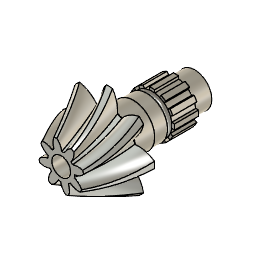
SanmitraGoswami helical bevel gear (Autodesk Fusion 360 design; units mm, degrees)
part number: 2025-10-19-15-40-55-736
Autodesk Fusion 360 part; units mm, degrees
sketch "Sketch2" plane through (0, 0, 0) normal (1, 0, 0) x (0, 1, 0)
  line L0 (5, 45) -> (5, 40)
  line L1 (5, 40) -> (45, 40)
  line L2 (45, 40) -> (45, 39)
  line L3 (45, 39) -> (70, 39)
  line L4 (70, 39) -> (70, 37)
  line L5 (80, 37) -> (125, 37)
  line L6 (125, 37) -> (125, 32)
  line L7 (125, 32) -> (160, 32)
  arc A0 (70, 37) -> (80, 37) centre (75, 37) ccw
  line L8 (5, 45) -> (0, 45)
  line L9 (0, 45) -> (0, 0)
  line L10 (0, 0) -> (160, 0)
  line L11 (160, 0) -> (160, 32)
  dimension "d3" = 5
  dimension "d4" = 1
  dimension "d5" = 2
  dimension "d6" = 5
  dimension "d8" = 40
  dimension "d9" = 25
  dimension "d10" = 35
  dimension "d11" = 10
  constraint perpendicular L0 L1
  constraint perpendicular L1 L2
  constraint perpendicular L2 L3
  constraint perpendicular L3 L4
  constraint perpendicular L4 L5
  constraint perpendicular L5 L6
  constraint perpendicular L0 L8
  constraint coincident L9.end L10.start
  constraint perpendicular L8 L9
  constraint perpendicular L9 L10
  constraint perpendicular L7 L11
  measures "d3" distance of L0.start L0.end
  measures "d4" distance of L1.end L2.end
  measures "d5" distance of L3.end L4.end
  measures "d6" distance of L5.end L6.end
  measures "d8" distance of L0.end L1.end
  measures "d9" distance of L2.end L3.end
  measures "d10" distance of L6.end L7.end
  measures "d11" diameter of A0
revolve "Revolve1" add sketch "Sketch2" angle 360 about axis through (0, 0, 0) along (0, 1, 0)
sketch "Sketch3" plane through (0, 0, 0) normal (0, -1, 0) x (1, 0, 0)
  circle A0 centre (0, 0) radius 45
  line L0 (0, 0) -> (0, -106.1302) construction
  line L1 (0, -106.1302) -> (0, 99.7894) construction
  arc A1 (-6, 84.788) -> (-15, 47.697) centre (39.6285, 54.079) ccw
  arc A2 (15, 47.697) -> (6, 84.788) centre (-39.6285, 54.079) ccw
  arc A3 (6, 84.788) -> (-6, 84.788) centre (0, 0) ccw
  arc A4 (-64.1968, 55.7115) -> (-44.3334, 23.1202) centre (-10.218, 66.2612) ccw
  arc A5 (-55.7115, 64.1968) -> (-64.1968, 55.7115) centre (0, 0) ccw
  arc A6 (-23.1202, 44.3334) -> (-55.7115, 64.1968) centre (-66.2612, 10.218) ccw
  arc A7 (-84.788, -6) -> (-47.697, -15) centre (-54.079, 39.6285) ccw
  arc A8 (-84.788, 6) -> (-84.788, -6) centre (0, 0) ccw
  arc A9 (-47.697, 15) -> (-84.788, 6) centre (-54.079, -39.6285) ccw
  arc A10 (-55.7115, -64.1968) -> (-23.1202, -44.3334) centre (-66.2612, -10.218) ccw
  arc A11 (-64.1968, -55.7115) -> (-55.7115, -64.1968) centre (0, 0) ccw
  arc A12 (-44.3334, -23.1202) -> (-64.1968, -55.7115) centre (-10.218, -66.2612) ccw
  arc A13 (6, -84.788) -> (15, -47.697) centre (-39.6285, -54.079) ccw
  arc A14 (-6, -84.788) -> (6, -84.788) centre (0, 0) ccw
  arc A15 (-15, -47.697) -> (-6, -84.788) centre (39.6285, -54.079) ccw
  arc A16 (64.1968, -55.7115) -> (44.3334, -23.1202) centre (10.218, -66.2612) ccw
  arc A17 (55.7115, -64.1968) -> (64.1968, -55.7115) centre (0, 0) ccw
  arc A18 (23.1202, -44.3334) -> (55.7115, -64.1968) centre (66.2612, -10.218) ccw
  arc A19 (84.788, 6) -> (47.697, 15) centre (54.079, -39.6285) ccw
  arc A20 (84.788, -6) -> (84.788, 6) centre (0, 0) ccw
  arc A21 (47.697, -15) -> (84.788, -6) centre (54.079, 39.6285) ccw
  arc A22 (55.7115, 64.1968) -> (23.1202, 44.3334) centre (66.2612, 10.218) ccw
  arc A23 (64.1968, 55.7115) -> (55.7115, 64.1968) centre (0, 0) ccw
  arc A24 (44.3334, 23.1202) -> (64.1968, 55.7115) centre (10.218, 66.2612) ccw
  arc A25 (-15, 47.697) -> (-23.1202, 44.3334) centre (0, 0) ccw
  arc A26 (-44.3334, 23.1202) -> (-47.697, 15) centre (0, 0) ccw
  arc A27 (-47.697, -15) -> (-44.3334, -23.1202) centre (0, 0) ccw
  arc A28 (-23.1202, -44.3334) -> (-15, -47.697) centre (0, 0) ccw
  arc A29 (15, -47.697) -> (23.1202, -44.3334) centre (0, 0) ccw
  arc A30 (44.3334, -23.1202) -> (47.697, -15) centre (0, 0) ccw
  arc A31 (47.697, 15) -> (44.3334, 23.1202) centre (0, 0) ccw
  arc A32 (23.1202, 44.3334) -> (15, 47.697) centre (0, 0) ccw
  dimension "d13" = 100
  dimension "d14" = 170
  dimension "d15" = 6
  dimension "d16" = 15
  dimension "d17" = 55
  dimension "d19" = 360
  constraint coincident A0.centre L0.start
  constraint vertical L0
  constraint parallel L0 L1
  constraint concentric A3 A26
  constraint coincident A1.end A26
  constraint symmetric L1 A1.start A2.end
  constraint symmetric L1 A1.end A2.start
  constraint symmetric L1 A1 A2
  constraint concentric A25 A26
  constraint concentric A26 A27
  constraint concentric A27 A28
  constraint concentric A28 A29
  constraint concentric A29 A30
  constraint concentric A30 A31
  constraint concentric A31 A32
  measures "d13" diameter of A26
  measures "d14" diameter of A3
  measures "d15" distance of L1 A1.start
  measures "d16" distance of L1 A1.end
  measures "d17" radius of A1
ref_plane "WorkPlane1" through (0, -45, 0) normal (0, -1, 0) x (1, 0, 0)
ref_plane "WorkPlane2" through (0, -140, 0) normal (0, -1, 0) x (-1, 0, 0)
sketch "Sketch5" plane through (0, -140, 0) normal (0, -1, 0) x (-1, 0, 0)
  arc A0 through (13.8701, -40.173, -50) (15.3515, -30.5933, -50) (13.4169, -21.0947, -50)
  arc A1 through (13.4169, -21.0947, -50) (15.219, -19.8338, -50) (16.9034, -18.4194, -50)
  arc A2 through (16.9034, -18.4194, -50) (25.5776, -22.7465, -50) (35.2143, -23.7951, -50)
  arc A3 through (35.2143, -23.7951, -50) (36.8061, -21.25, -50) (38.2143, -18.5989, -50)
  arc A4 through (38.2143, -18.5989, -50) (32.4879, -10.7776, -50) (24.4034, -5.429, -50)
  arc A5 through (24.4034, -5.429, -50) (24.7861, -3.2632, -50) (24.977, -1.072, -50)
  arc A6 through (24.977, -1.072, -50) (34.1703, 2.0019, -50) (41.7259, 8.0746, -50)
  arc A7 through (41.7259, 8.0746, -50) (41.0518, 10.9998, -50) (40.173, 13.8701, -50)
  arc A8 through (40.173, 13.8701, -50) (30.5933, 15.3515, -50) (21.0947, 13.4169, -50)
  arc A9 through (21.0947, 13.4169, -50) (19.8338, 15.219, -50) (18.4194, 16.9034, -50)
  arc A10 through (18.4194, 16.9034, -50) (22.7465, 25.5776, -50) (23.7951, 35.2143, -50)
  arc A11 through (23.7951, 35.2143, -50) (21.25, 36.8061, -50) (18.5989, 38.2143, -50)
  arc A12 through (18.5989, 38.2143, -50) (10.7776, 32.4879, -50) (5.429, 24.4034, -50)
  arc A13 through (5.429, 24.4034, -50) (3.2632, 24.7861, -50) (1.072, 24.977, -50)
  arc A14 through (1.072, 24.977, -50) (-2.0019, 34.1703, -50) (-8.0746, 41.7259, -50)
  arc A15 through (-8.0746, 41.7259, -50) (-10.9998, 41.0518, -50) (-13.8701, 40.173, -50)
  arc A16 through (-13.8701, 40.173, -50) (-15.3515, 30.5933, -50) (-13.4169, 21.0947, -50)
  arc A17 through (-13.4169, 21.0947, -50) (-15.219, 19.8338, -50) (-16.9034, 18.4194, -50)
  arc A18 through (-16.9034, 18.4194, -50) (-25.5776, 22.7465, -50) (-35.2143, 23.7951, -50)
  arc A19 through (-35.2143, 23.7951, -50) (-36.8061, 21.25, -50) (-38.2143, 18.5989, -50)
  arc A20 through (-38.2143, 18.5989, -50) (-32.4879, 10.7776, -50) (-24.4034, 5.429, -50)
  arc A21 through (-24.4034, 5.429, -50) (-24.7861, 3.2632, -50) (-24.977, 1.072, -50)
  arc A22 through (-24.977, 1.072, -50) (-34.1703, -2.0019, -50) (-41.7259, -8.0746, -50)
  arc A23 through (-41.7259, -8.0746, -50) (-41.0518, -10.9998, -50) (-40.173, -13.8701, -50)
  arc A24 through (-40.173, -13.8701, -50) (-30.5933, -15.3515, -50) (-21.0947, -13.4169, -50)
  arc A25 through (-21.0947, -13.4169, -50) (-19.8338, -15.219, -50) (-18.4194, -16.9034, -50)
  arc A26 through (-18.4194, -16.9034, -50) (-22.7465, -25.5776, -50) (-23.7951, -35.2143, -50)
  arc A27 through (-23.7951, -35.2143, -50) (-21.25, -36.8061, -50) (-18.5989, -38.2143, -50)
  arc A28 through (-18.5989, -38.2143, -50) (-10.7776, -32.4879, -50) (-5.429, -24.4034, -50)
  arc A29 through (-5.429, -24.4034, -50) (-3.2632, -24.7861, -50) (-1.072, -24.977, -50)
  arc A30 through (8.0746, -41.7259, -50) (10.9998, -41.0518, -50) (13.8701, -40.173, -50)
  arc A31 through (-1.072, -24.977, -50) (2.0019, -34.1703, -50) (8.0746, -41.7259, -50)
ref_plane "WorkPlane3" through (0, -45, 0) normal (0, -1, 0) x (1, 0, 0)
sketch "Sketch6" plane through (0, -45, 0) normal (0, -1, 0) x (-1, 0, 0)
  arc A0 (8.1436, -36.6051) -> (27.8984, -57.3214) centre (46.0191, -20.2646) ccw
  arc A1 (27.8984, -57.3214) -> (35.6926, -52.8214) centre (0, 0) ccw
  arc A2 (35.6926, -52.8214) -> (27.6291, -25.3551) centre (-5.4598, -49.986) ccw
  arc A3 (27.6291, -25.3551) -> (31.6421, -20.1253) centre (0, 0) ccw
  arc A4 (31.6421, -20.1253) -> (60.2595, -20.8052) centre (46.8697, 18.2111) ccw
  arc A5 (60.2595, -20.8052) -> (62.5889, -12.1119) centre (0, 0) ccw
  arc A6 (62.5889, -12.1119) -> (37.4655, 1.608) centre (31.4848, -39.2061) ccw
  arc A7 (37.4655, 1.608) -> (36.6051, 8.1436) centre (0, 0) ccw
  arc A8 (36.6051, 8.1436) -> (57.3214, 27.8984) centre (20.2646, 46.0191) ccw
  arc A9 (57.3214, 27.8984) -> (52.8214, 35.6926) centre (0, 0) ccw
  arc A10 (52.8214, 35.6926) -> (25.3551, 27.6291) centre (49.986, -5.4598) ccw
  arc A11 (25.3551, 27.6291) -> (20.1253, 31.6421) centre (0, 0) ccw
  arc A12 (20.1253, 31.6421) -> (20.8052, 60.2595) centre (-18.2111, 46.8697) ccw
  arc A13 (20.8052, 60.2595) -> (12.1119, 62.5889) centre (0, 0) ccw
  arc A14 (12.1119, 62.5889) -> (-1.608, 37.4655) centre (39.2061, 31.4848) ccw
  arc A15 (-1.608, 37.4655) -> (-8.1436, 36.6051) centre (0, 0) ccw
  arc A16 (-8.1436, 36.6051) -> (-27.8984, 57.3214) centre (-46.0191, 20.2646) ccw
  arc A17 (-27.8984, 57.3214) -> (-35.6926, 52.8214) centre (0, 0) ccw
  arc A18 (-35.6926, 52.8214) -> (-27.6291, 25.3551) centre (5.4598, 49.986) ccw
  arc A19 (-27.6291, 25.3551) -> (-31.6421, 20.1253) centre (0, 0) ccw
  arc A20 (-31.6421, 20.1253) -> (-60.2595, 20.8052) centre (-46.8697, -18.2111) ccw
  arc A21 (-60.2595, 20.8052) -> (-62.5889, 12.1119) centre (0, 0) ccw
  arc A22 (-62.5889, 12.1119) -> (-37.4655, -1.608) centre (-31.4848, 39.2061) ccw
  arc A23 (-37.4655, -1.608) -> (-36.6051, -8.1436) centre (0, 0) ccw
  arc A24 (-36.6051, -8.1436) -> (-57.3214, -27.8984) centre (-20.2646, -46.0191) ccw
  arc A25 (-57.3214, -27.8984) -> (-52.8214, -35.6926) centre (0, 0) ccw
  arc A26 (-52.8214, -35.6926) -> (-25.3551, -27.6291) centre (-49.986, 5.4598) ccw
  arc A27 (-25.3551, -27.6291) -> (-20.1253, -31.6421) centre (0, 0) ccw
  arc A28 (-20.1253, -31.6421) -> (-20.8052, -60.2595) centre (18.2111, -46.8697) ccw
  arc A29 (-20.8052, -60.2595) -> (-12.1119, -62.5889) centre (0, 0) ccw
  arc A30 (1.608, -37.4655) -> (8.1436, -36.6051) centre (0, 0) ccw
  arc A31 (-12.1119, -62.5889) -> (1.608, -37.4655) centre (-39.2061, -31.4848) ccw
loft "Loft1" add profiles "Sketch5", "Sketch6", "Sketch3" section 1 contours A0 A1 A2 A3 A4 A5 A6 A7 A8 A9 A10 A11 A12 A13 A14 A15 A16 A17 A18 A19 A20 A21 A22 A23 A24 A25 A26 A27 A28 A29 A30 A31 in plane through (0, -90, 0) normal (0, -1, 0) section 2 section 3
sketch "Sketch7" plane through (0, 125, 0) normal (0, 1, 0) x (-1, 0, 0)
  circle A0 centre (0, 0) radius 37
  circle A1 centre (0, 0) radius 32
  line L0 (5, 42) -> (-5, 42)
  line L1 (-5, 42) -> (-5, 37)
  line L2 (-5, 37) -> (5, 37)
  line L3 (5, 37) -> (5, 42)
  line L4 (5, 42) -> (-5, 37) construction
  line L5 (-5, 42) -> (5, 37) construction
  line L6 (-5, 37) -> (-5, 36.6606)
  line L7 (5, 37) -> (5, 36.6606)
  point P0 (0, 39.5)
  dimension "d23" = 10
  dimension "d24" = 5
  constraint horizontal L0
  constraint perpendicular L0 L1
  constraint parallel L0 L2
  constraint parallel L1 L3
  constraint coincident L4 P0
  constraint coincident L5 P0
  constraint tangent A0 L2
  constraint coincident A0 L6.end
  constraint perpendicular L2 L6
  constraint coincident A0 L7.end
  constraint perpendicular L2 L7
  measures "d23" distance of L1.end L2.end
  measures "d24" distance of L0.end L1.end
extrude "Extrude1" add sketch "Sketch7" against normal blind 45 contours A0 L2 L7 | A0 L2 L6 | L0 L1 L2 L3
pattern_circular "C-Pattern1" count 12 over 360 about axis through (0, 160, 0) along (0, 1, 0) of "Extrude1"
hole "Hole1" at (0, 160, 0) direction (0, -1, 0) diameter 35 depth 300 tip angle 180
